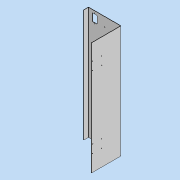
# Autodesk Inventor part: Controller_Panel
Saved by Autodesk Inventor 2020 (Build 240168000, 168)
## iProperties
Created: 2021-05-17
Part Number: Controller_Panel
Material: 一般
Document SubType Name: Sheet Metal
Designer: ken113
Density: 1 g/cm^3
Sheet Metal Rule: Default_mm
Appearance: 既定
Author: ken113
Autodesk Inventor part; units mm, degrees
ref_plane "YZ Plane" through (0, 0, 0) normal (1, 0, 0) x (0, 1, 0)
ref_plane "XZ Plane" through (0, 0, 0) normal (0, 1, 0) x (-1, 0, 0)
ref_plane "XY Plane" through (0, 0, 0) normal (0, 0, 1) x (1, 0, 0)
sketch "スケッチ1" plane through (0, 0, 0) normal (0, 0, 1) x (1, 0, 0)
  line L0 (100, -345) -> (-100, -345)
  line L1 (-100, -345) -> (-100, 345)
  line L2 (-100, 345) -> (100, 345)
  line L3 (100, 345) -> (100, -345)
  line L4 (100, -345) -> (-100, 345) construction
  line L5 (-100, -345) -> (100, 345) construction
  point P0 (0, 0)
  dimension "d0" = 200
  dimension "d1" = 690
  measures "d0" distance of L1.end L2.end
  measures "d1" distance of L0.end L1.end
extrude "プレート1" add sketch "スケッチ1" along normal blind 2
sketch "スケッチ2" plane through (-98, -345, 0) normal (-1, 0, 0) x (0, -1, 0)
  line L0 (-690, 0) -> (0, 0)
  line L1 (0, 0) -> (0, 30)
  line L2 (0, 30) -> (-690, 30)
  line L3 (-690, 30) -> (-690, 0)
  constraints: 6 end point, 1 horizontal, 1 perpendicular, 1 vertical
edge flange "フランジ1" height 30 angle 90 thickness 2 bend radius 2 thickness toward (-1, 0, 0) relief straight relief width 2 relief depth 1 edges at (-100, 0, 2) wall of the first edge with corners at (-98, 345, 0) (-98, -345, 0) (-98, -345, 30) (-98, 345, 30)
bend "曲げ1"
corner "コーナー1"
sketch "スケッチ6" plane through (0, 0, 0) normal (0, 0, -1) x (-1, 0, 0)
  line L0 (46, 281.5) -> (74, 281.5)
  line L1 (74, 281.5) -> (74, 328.5)
  line L2 (74, 328.5) -> (46, 328.5)
  line L3 (46, 328.5) -> (46, 281.5)
  line L4 (46, 281.5) -> (74, 328.5) construction
  line L5 (74, 281.5) -> (46, 328.5) construction
  line L6 (96, 345) -> (-100, 345) projected
  line L7 (100, 345) -> (100, -345) projected
  point P0 (0, 0)
  point P1 (60, 305)
  dimension "d40" = 28
  dimension "d41" = 47
  dimension "d83" = 40
  dimension "d84" = 40
  constraints: 12 end point, 2 midpoint, 2 parallel, 1 horizontal, 1 perpendicular
  measures "d40" distance of L2.end L1.end
  measures "d41" distance of L1.end L0.end
  measures "d83" distance from line of L6 point (60, 305)
  measures "d84" distance from line of L7 point (60, 305)
extrude "押し出し2" cut sketch "スケッチ6" against normal blind 10
sketch "スケッチ7" plane through (0, 0, 0) normal (0, 0, -1) x (-1, 0, 0)
  line L0 (46, 281.5) -> (46, 328.5) projected
  line L1 (46, 328.5) -> (74, 328.5) projected
  line L2 (74, 328.5) -> (74, 281.5) projected
  line L3 (74, 281.5) -> (46, 281.5) projected
  line L4 (96, -345) -> (96, 345) projected
  line L5 (74, 328.5) -> (74, 281.5) projected
  line L6 (46, 328.5) -> (74, 328.5) projected
  line L7 (-100, -345) -> (96, -345) projected
  line L8 (96, 345) -> (-100, 345) projected
  line L9 (-100, 345) -> (-100, -345) projected
  line L10 (74, 281.5) -> (46, 281.5) projected
  point P0 (0, 0)
  point P1 (60, 333)
  point P2 (60, 277)
  point P3 (74, 305)
  point P4 (74, 305)
  point P5 (60, 281.5)
  point P6 (60, 281.5)
  dimension "d87" = 56
  dimension "d88" = 28
  constraints: 4 midpoint, 2 vertical alignment
  measures "d87" distance of point (60, 333) point (60, 277)
  measures "d88" vertical distance of point (74, 305) point (60, 277)
hole "穴2" at (-60, 333, 0) at (-60, 277, 0) direction (0, 0, 1) diameter 3.2 end through all
fillet "フィレット1" radius 2 4 edges at (-46, 281.5, 1) (-74, 281.5, 1) (-46, 328.5, 1) (-74, 328.5, 1)
sketch "スケッチ9" plane through (98, 345, 0) normal (1, 0, 0) x (0, 1, 0)
  line L0 (-690, 0) -> (0, 0)
  line L1 (0, 0) -> (0, 182)
  line L2 (0, 182) -> (-690, 182)
  line L3 (-690, 182) -> (-690, 0)
  constraints: 6 end point, 1 horizontal, 1 perpendicular, 1 vertical
edge flange "フランジ3" height 182 angle 90 thickness 2 bend radius 2 thickness toward (1, 0, 0) relief straight relief width 2 relief depth 1 edges at (100, 0, 2) wall of the first edge with corners at (98, -345, 0) (98, 345, 0) (98, 345, 182) (98, -345, 182)
bend "曲げ3"
corner "コーナー3"
sketch "スケッチ10" plane through (0, 0, 0) normal (0, 0, -1) x (-1, 0, 0)
  line L0 (-96, 345) -> (-96, -345) projected
  line L1 (-96, -345) -> (96, -345) projected
  line L2 (96, -345) -> (96, 345) projected
  line L3 (96, 345) -> (-96, 345) projected
  line L4 (74, 326.5) -> (74, 283.5) projected
  arc A0 (72, 281.5) -> (74, 283.5) centre (72, 283.5) ccw projected
  line L5 (72, 281.5) -> (48, 281.5) projected
  arc A1 (46, 283.5) -> (48, 281.5) centre (48, 283.5) ccw projected
  line L6 (46, 283.5) -> (46, 326.5) projected
  arc A2 (48, 328.5) -> (46, 326.5) centre (48, 326.5) ccw projected
  line L7 (48, 328.5) -> (72, 328.5) projected
  arc A3 (74, 326.5) -> (72, 328.5) centre (72, 326.5) ccw projected
  circle A4 centre (60, 277) radius 1.6 projected
  circle A5 centre (60, 333) radius 1.6 projected
  line L8 (-1, 140) -> (-51, 140)
  line L9 (-51, 140) -> (-51, 290)
  line L10 (-51, 290) -> (-1, 290)
  line L11 (-1, 290) -> (-1, 140)
  line L12 (-1, 140) -> (-51, 290) construction
  line L13 (-51, 140) -> (-1, 290) construction
  point P0 (0, 0)
  point P1 (-26, 215)
  dimension "d89" = 50
  dimension "d90" = 150
  dimension "d91" = 70
  dimension "d92" = 130
  constraints: 12 end point, 2 midpoint, 2 parallel, 1 horizontal, 1 perpendicular
  measures "d89" distance of L9.end L10.end
  measures "d90" distance of L8.end L9.end
  measures "d91" distance from line of point (-26, 215) L0
  measures "d92" distance from line of point (-26, 215) L3
hole "穴4" at (51, 140, 0) at (1, 140, 0) at (1, 290, 0) at (51, 290, 0) direction (0, 0, 1) diameter 4.2 depth 2 tip angle 118
sketch "スケッチ11" plane through (0, 0, 2) normal (0, 0, 1) x (1, 0, 0)
  circle A0 centre (1, 290) radius 2.1 projected
  circle A1 centre (51, 140) radius 2.1 projected
  circle A2 centre (1, 140) radius 2.1 projected
  circle A3 centre (51, 290) radius 2.1 projected
  line L0 (96, -345) -> (96, 345) projected
  line L1 (-96, 345) -> (96, 345) projected
  line L2 (-96, 345) -> (-96, -345) projected
  line L3 (96, -345) -> (-96, -345) projected
  circle A4 centre (-60, 333) radius 1.6 projected
  circle A5 centre (-60, 277) radius 1.6 projected
  line L4 (-74, 283.5) -> (-74, 326.5) projected
  arc A6 (-72, 328.5) -> (-74, 326.5) centre (-72, 326.5) ccw projected
  line L5 (-72, 328.5) -> (-48, 328.5) projected
  arc A7 (-46, 326.5) -> (-48, 328.5) centre (-48, 326.5) ccw projected
  line L6 (-46, 326.5) -> (-46, 283.5) projected
  arc A8 (-48, 281.5) -> (-46, 283.5) centre (-48, 283.5) ccw projected
  line L7 (-48, 281.5) -> (-72, 281.5) projected
  arc A9 (-74, 283.5) -> (-72, 281.5) centre (-72, 283.5) ccw projected
  point P0 (0, 0)
  point P1 (46, 65)
  point P2 (46, -5)
  point P3 (46, -75)
  point P4 (46, -145)
  dimension "d102" = 70
  dimension "d107" = 50
  dimension "d108" = 280
  constraints: 1 vertical, 3 other
  measures "d102" distance of point (46, 65) point (46, -5)
  measures "d107" distance from line of point (46, 65) L0
  measures "d108" distance from line of L1 point (46, 65)
hole "穴5" at (46, 65, 2) at (46, -5, 2) at (46, -75, 2) at (46, -145, 2) direction (0, 0, -1) diameter 4.2 depth 2 tip angle 118
sketch "スケッチ12" plane through (0, 0, 2) normal (0, 0, 1) x (1, 0, 0)
  circle A0 centre (46, -75) radius 2.1 projected
  circle A1 centre (46, 65) radius 2.1 projected
  circle A2 centre (46, -5) radius 2.1 projected
  circle A3 centre (46, -145) radius 2.1 projected
  circle A4 centre (1, 290) radius 2.1 projected
  circle A5 centre (51, 140) radius 2.1 projected
  circle A6 centre (1, 140) radius 2.1 projected
  circle A7 centre (51, 290) radius 2.1 projected
  line L0 (96, -345) -> (96, 345) projected
  line L1 (-96, 345) -> (96, 345) projected
  line L2 (-96, 345) -> (-96, -345) projected
  line L3 (96, -345) -> (-96, -345) projected
  circle A8 centre (-60, 333) radius 1.6 projected
  circle A9 centre (-60, 277) radius 1.6 projected
  line L4 (-74, 283.5) -> (-74, 326.5) projected
  arc A10 (-72, 328.5) -> (-74, 326.5) centre (-72, 326.5) ccw projected
  line L5 (-72, 328.5) -> (-48, 328.5) projected
  arc A11 (-46, 326.5) -> (-48, 328.5) centre (-48, 326.5) ccw projected
  line L6 (-46, 326.5) -> (-46, 283.5) projected
  arc A12 (-48, 281.5) -> (-46, 283.5) centre (-48, 283.5) ccw projected
  line L7 (-48, 281.5) -> (-72, 281.5) projected
  arc A13 (-74, 283.5) -> (-72, 281.5) centre (-72, 283.5) ccw projected
  point P0 (0, 0)
  point P1 (76, -315)
  point P2 (-39, -315)
  point P3 (76, -275)
  point P4 (-39, -275)
  point P5 (76, -235)
  point P6 (-39, -235)
  dimension "d116" = 115
  dimension "d119" = 40
  dimension "d124" = 20
  dimension "d125" = 580
  constraints: 1 horizontal alignment, 1 vertical, 4 other
  measures "d116" distance of point (76, -315) point (-39, -315)
  measures "d119" distance of point (76, -315) point (76, -275)
  measures "d124" distance from line of point (76, -235) L0
  measures "d125" distance from line of L1 point (76, -235)
hole "穴6" at (76, -315, 2) at (-39, -315, 2) at (76, -275, 2) at (-39, -275, 2) at (76, -235, 2) at (-39, -235, 2) direction (0, 0, -1) diameter 4.2 depth 2 tip angle 118
sketch "スケッチ13" plane through (100, -345, 182) normal (1, 0, 0) x (0, 0, -1)
  line L0 (7.5, 540) -> (62.5, 540)
  line L1 (62.5, 540) -> (62.5, 590)
  line L2 (62.5, 590) -> (7.5, 590)
  line L3 (7.5, 590) -> (7.5, 540)
  line L4 (7.5, 540) -> (62.5, 590) construction
  line L5 (62.5, 540) -> (7.5, 590) construction
  line L6 (7.5, 100) -> (62.5, 100)
  line L7 (62.5, 100) -> (62.5, 150)
  line L8 (62.5, 150) -> (7.5, 150)
  line L9 (7.5, 150) -> (7.5, 100)
  line L10 (7.5, 100) -> (62.5, 150) construction
  line L11 (62.5, 100) -> (7.5, 150) construction
  line L12 (0, 0) -> (0, 690) projected
  line L13 (178, 0) -> (0, 0) projected
  line L14 (0, 690) -> (178, 690) projected
  point P0 (182, 345)
  point P1 (35, 565)
  point P2 (35, 125)
  point P3 (35, 565)
  point P4 (35, 125)
  dimension "d133" = 55
  dimension "d134" = 50
  dimension "d135" = 55
  dimension "d136" = 50
  dimension "d137" = 7.5
  dimension "d138" = 100
  dimension "d139" = 100
  constraints: 24 end point, 6 midpoint, 4 parallel, 2 horizontal, 2 perpendicular, 1 vertical alignment
  measures "d133" distance of L2.end L1.end
  measures "d134" distance of L1.end L0.end
  measures "d135" distance of L8.end L7.end
  measures "d136" distance of L7.end L6.end
  measures "d137" distance between parallel lines of L9 L12
  measures "d138" distance between parallel lines of L6 L13
  measures "d139" distance between parallel lines of L14 L2
hole "穴7" at (100, 245, 174.5) at (100, 195, 174.5) at (100, 195, 119.5) at (100, 245, 119.5) at (100, -195, 174.5) at (100, -245, 174.5) at (100, -245, 119.5) at (100, -195, 119.5) direction (-1, 0, 0) diameter 4.134 depth 14.2 tip angle 118 thread size "M5x0.8" class "6H" standard "ISO Metric profile"
equation "\"d53\" = Thickness"
equation "\"d98\" = Thickness"
equation "\"d114\" = Thickness"
equation "\"d131\" = Thickness"
equation "\"d2\" = Thickness"
equation "\"d3\" = BendReliefWidth"
equation "\"d4\" = BendReliefDepth"
equation "\"d5\" = MinimumRemnant"
equation "\"d6\" = TransitionRadius"
equation "\"d9\" = BendRadius"
equation "\"d10\" = CornerReliefSize"
equation "\"d11\" = GapSize"
equation "\"d12\" = JacobiRadiusSize"
equation "\"d73\" = BendReliefWidth"
equation "\"d74\" = BendReliefDepth"
equation "\"d75\" = MinimumRemnant"
equation "\"d76\" = TransitionRadius"
equation "\"d79\" = BendRadius"
equation "\"d80\" = CornerReliefSize"
equation "\"d81\" = GapSize"
equation "\"d82\" = JacobiRadiusSize"
equation "\"BendRadius\" = Thickness"
equation "\"BendReliefWidth\" = Thickness"
equation "\"BendReliefDepth\" = 0.5 * Thickness"
equation "\"CornerReliefSize\" = 4 * Thickness"
equation "\"MinimumRemnant\" = 2 * Thickness"
equation "\"TransitionRadius\" = BendRadius"
equation "\"JacobiRadiusSize\" = BendRadius"
equation "\"GapSize\" = Thickness"
equation "\"Thickness\" = 2"
